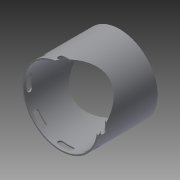
# Autodesk Inventor part: Colossus_7kW_Rotor_body
Saved by Autodesk Inventor 2014 (Build 180170000, 170)
## iProperties
Created: 2014-11-23
Part Number: Colossus_7kW_Rotor_body
Material: Générique
Document SubType Name: Modeling
Designer: Yann
Density: 1 g/cm^3
Appearance: Par défaut
Author: Yann
Autodesk Inventor part; units mm, degrees
ref_plane "YZ Plane" through (0, 0, 0) normal (1, 0, 0) x (0, 1, 0)
ref_plane "XZ Plane" through (0, 0, 0) normal (0, 1, 0) x (-1, 0, 0)
ref_plane "XY Plane" through (0, 0, 0) normal (0, 0, 1) x (1, 0, 0)
sketch "Esquisse1" plane through (0, 0, 0) normal (0, 1, 0) x (-1, 0, 0)
  line L0 (0, -80.29) -> (0, 80.29) construction
  line L1 (-80.29, 0) -> (80.29, 0) construction
  circle A0 centre (0, 0) radius 57.35
  circle A1 centre (0, 0) radius 55.35
  circle A2 centre (0, 0) radius 16 construction
  circle A3 centre (0, 0) radius 57.35 construction
  dimension "d0" = 2
  constraints: 2 centre point, 2 coincident, 1 concentric
  measures "d0" radial gap between concentric circles of A0 A1
extrude "Extrusion1" add sketch "Esquisse1" against normal blind 89.3
sketch "Esquisse2" plane through (0, 0, 0) normal (1, 0, 0) x (0, 1, 0)
  line L0 (-80.3, 18.5) -> (-80.3, -18.5) construction
  line L1 (-85.3, 18.5) -> (-85.3, -18.5)
  line L2 (-75.3, -18.5) -> (-75.3, 18.5)
  arc A0 (-75.3, 18.5) -> (-85.3, 18.5) centre (-80.3, 18.5) ccw
  arc A1 (-85.3, -18.5) -> (-75.3, -18.5) centre (-80.3, -18.5) ccw
  line L3 (-89.3, 57.35) -> (-89.3, -57.35) construction
  line L4 (-81.6, 0) -> (13.6, 0) construction
  point P0 (0, 0)
  point P1 (-80.3, 0)
  dimension "d3" = 4
  dimension "d4" = 5
  dimension "d5" = 37
  constraints: 8 end point, 4 point on circle, 4 tangent, 2 centre point, 2 parallel, 1 midpoint, 1 symmetric about line
  measures "d3" distance between parallel lines of L3 L1
  measures "d4" radius of A0
  measures "d5" distance of L0.start L0.end
extrude "Extrusion2" cut sketch "Esquisse2" against normal blind 68
pattern_circular "Réseau circulaire1" count 6 over 360 about axis through (0, -10, 0) along (0, 1, 0) of "Extrusion2"
